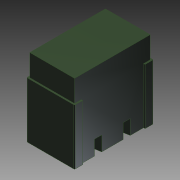
# Autodesk Inventor part: MB2011-body
Saved by Autodesk Inventor 2015 (Build 190159000, 159)
## iProperties
Category: PARTsolutions
Company: NKKSWITCHES
Created: 2015-01-04
Part Number: MB2011-body
Catalog Web Link: www.cadenas.de
Description: MB2000 Series - Bushing Mount Miniature Pushbuttons -body-
Vendor: NKKSWITCHES
Document SubType Name: Modeling
Designer: PARTuser1
Manufacturer: NKKSWITCHES
Mass: 1.21725 g
Surface Area: 7.52503 cm^2
Volume: 1.21725 cm^3
Density: 1 g/cm^3
Material: Generic
Appearance: PSOLRGB-79-119-66
PSOL_IDENT_0: {$CADENAS_DATA\23d-libs\nkkswitches\pushbuttons\mb2000\parts\mb2000_body.prj},223 {VTYP=3D},{NB=MB20
PSOL_IDENT_1: 11-body},{LINA=MB2011-body},{NN=MB2000 Series - Bushing Mount Miniature Pushbuttons -body},{DATE=21.
PSOL_IDENT_2: 11.2014 08:56:24},{GEOMDATE=14.04.2009 08:35:00},{VERSION=},{LINEID=10},{LINESUBID=-1},{WBVAR=PLSCRC
PSOL_IDENT_3: TS}  {NB=MB2011-body},{LINA=MB2011-body},{KT=DUMMY},{PN=MB2011},{SRS=MB},{PLSCRCTS=2011}
SUPPLIER: NKKSWITCHES
ARTICLENO: MB2011-body
BOMINFO: MB2011-body
CREATOR: CADENAS GmbH
Title: MB2011-body
Author: Cadenas PARTsolutions
Autodesk Inventor part; units mm, degrees
sketch "Sketch_1" plane through (0, 0, 0) normal (0, 1, 0) x (-1, 0, 0)
  line L0 (3.9497, 5.1435) -> (3.9497, 6.3754)
  arc A0 (3.9497, 6.3754) -> (3.8227, 6.5024) centre (3.8227, 6.3754) ccw
  line L1 (3.8227, 6.5024) -> (-3.8227, 6.5024)
  arc A1 (-3.8227, 6.5024) -> (-3.9497, 6.3754) centre (-3.8227, 6.3754) ccw
  line L2 (-3.9497, 6.3754) -> (-3.9497, 5.1435)
  line L3 (-3.9497, 5.1435) -> (-3.6957, 5.1435)
  line L4 (-3.6957, 5.1435) -> (-3.6957, 2.9397)
  line L5 (-3.6957, 2.9397) -> (-2.6797, 2.7606)
  line L6 (-2.6797, 2.7606) -> (-2.6797, 1.9384)
  line L7 (-2.6797, 1.9384) -> (-3.6957, 1.7593)
  line L8 (-3.6957, 1.7593) -> (-3.6957, -1.7593)
  line L9 (-3.6957, -1.7593) -> (-2.6797, -1.9384)
  line L10 (-2.6797, -1.9384) -> (-2.6797, -2.7606)
  line L11 (-2.6797, -2.7606) -> (-3.6957, -2.9397)
  line L12 (-3.6957, -2.9397) -> (-3.6957, -5.1435)
  line L13 (-3.6957, -5.1435) -> (-3.9497, -5.1435)
  line L14 (-3.9497, -5.1435) -> (-3.9497, -6.3754)
  arc A2 (-3.9497, -6.3754) -> (-3.8227, -6.5024) centre (-3.8227, -6.3754) ccw
  line L15 (-3.8227, -6.5024) -> (3.8227, -6.5024)
  arc A3 (3.8227, -6.5024) -> (3.9497, -6.3754) centre (3.8227, -6.3754) ccw
  line L16 (3.9497, -6.3754) -> (3.9497, -5.1435)
  line L17 (3.9497, -5.1435) -> (3.6957, -5.1435)
  line L18 (3.6957, -5.1435) -> (3.6957, -2.9397)
  line L19 (3.6957, -2.9397) -> (2.6797, -2.7606)
  line L20 (2.6797, -2.7606) -> (2.6797, -1.9384)
  line L21 (2.6797, -1.9384) -> (3.6957, -1.7593)
  line L22 (3.6957, -1.7593) -> (3.6957, 1.7593)
  line L23 (3.6957, 1.7593) -> (2.6797, 1.9384)
  line L24 (2.6797, 1.9384) -> (2.6797, 2.7606)
  line L25 (2.6797, 2.7606) -> (3.6957, 2.9397)
  line L26 (3.6957, 2.9397) -> (3.6957, 5.1435)
  line L27 (3.6957, 5.1435) -> (3.9497, 5.1435)
  constraints: 56 end point, 8 point on circle, 4 centre point
extrude "Extrusion1" add sketch "Sketch_1" against normal blind 9.1694
sketch "Sketch_2" plane through (0, 0, 0) normal (0, 1, 0) x (-1, 0, 0)
  line L0 (3.6957, 6.2484) -> (-3.6957, 6.2484)
  line L1 (-3.6957, 6.2484) -> (-3.6957, -6.2484)
  line L2 (-3.6957, -6.2484) -> (3.6957, -6.2484)
  line L3 (3.6957, -6.2484) -> (3.6957, 6.2484)
  constraints: 8 end point
extrude "Extrusion2" add sketch "Sketch_2" along normal blind 3.5814
sketch "Sketch_28" plane through (0, 0, 0) normal (0, 1, 0) x (-1, 0, 0)
  line L0 (3.6957, 6.2484) -> (-3.6957, 6.2484)
  line L1 (-3.6957, 6.2484) -> (-3.6957, -6.2484)
  line L2 (-3.6957, -6.2484) -> (3.6957, -6.2484)
  line L3 (3.6957, -6.2484) -> (3.6957, 6.2484)
  constraints: 8 end point
extrude "Extrusion3" add sketch "Sketch_28" against normal blind 6.7564
sketch "Sketch_9" plane through (0, -9.1694, 0) normal (0, 1, 0) x (1, 0, 0)
  arc A0 (-2.286, 2.3194) -> (-2.032, 2.0654) centre (-2.032, 2.3194) ccw
  line L0 (-2.032, 2.0654) -> (2.032, 2.0654)
  arc A1 (2.032, 2.0654) -> (2.286, 2.3194) centre (2.032, 2.3194) ccw
  line L1 (2.286, 2.3194) -> (2.286, 2.3796)
  arc A2 (2.286, 2.3796) -> (2.032, 2.6336) centre (2.032, 2.3796) ccw
  line L2 (2.032, 2.6336) -> (-2.032, 2.6336)
  arc A3 (-2.032, 2.6336) -> (-2.286, 2.3796) centre (-2.032, 2.3796) ccw
  line L3 (-2.286, 2.3796) -> (-2.286, 2.3194)
  constraints: 8 end point, 8 point on circle, 4 centre point
extrude "Extrusion4" add sketch "Sketch_9" against normal blind 0.508
sketch "Sketch_10" plane through (0, -9.1694, 0) normal (0, 1, 0) x (1, 0, 0)
  line L0 (-2.286, -2.3194) -> (-2.286, -2.3796)
  arc A0 (-2.286, -2.3796) -> (-2.032, -2.6336) centre (-2.032, -2.3796) ccw
  line L1 (-2.032, -2.6336) -> (2.032, -2.6336)
  arc A1 (2.032, -2.6336) -> (2.286, -2.3796) centre (2.032, -2.3796) ccw
  line L2 (2.286, -2.3796) -> (2.286, -2.3194)
  arc A2 (2.286, -2.3194) -> (2.032, -2.0654) centre (2.032, -2.3194) ccw
  line L3 (2.032, -2.0654) -> (-2.032, -2.0654)
  arc A3 (-2.032, -2.0654) -> (-2.286, -2.3194) centre (-2.032, -2.3194) ccw
  constraints: 8 end point, 8 point on circle, 4 centre point
extrude "Extrusion5" add sketch "Sketch_10" against normal blind 0.508
ref_plane "to_bm_terminals_XY" through (0, -8.9154, 0) normal (0, -1, 0) x (1, 0, 0)
ref_plane "to_bm_terminals_YZ" through (0, -8.9154, 0) normal (1, 0, 0) x (0, 0, 1)
ref_plane "to_bm_terminals_ZX" through (0, -8.9154, 0) normal (0, 0, 1) x (0, -1, 0)
ref_plane "to_bodycover_XY" through (0, 3.5814, 0) normal (0, -1, 0) x (1, 0, 0)
ref_plane "to_bodycover_YZ" through (0, 3.5814, 0) normal (1, 0, 0) x (0, 0, 1)
ref_plane "to_bodycover_ZX" through (0, 3.5814, 0) normal (0, 0, 1) x (0, -1, 0)
ref_plane "to_dummy_XY" through (0, 0, 0) normal (0, -1, 0) x (1, 0, 0)
ref_plane "to_dummy_YZ" through (0, 0, 0) normal (1, 0, 0) x (0, 0, 1)
ref_plane "to_dummy_ZX" through (0, 0, 0) normal (0, 0, 1) x (0, -1, 0)
body "Solid1"
